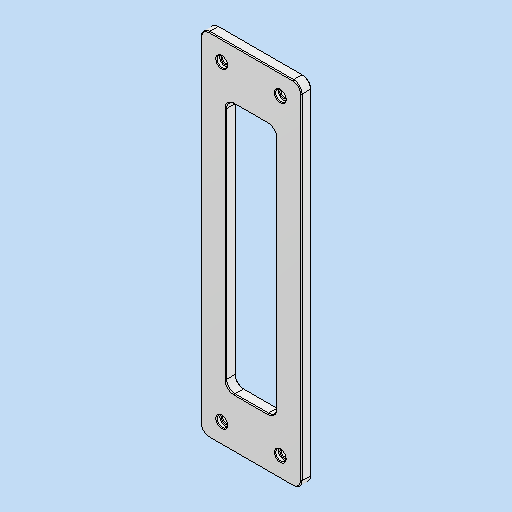
# Autodesk Inventor part: tc-top-bar
Saved by Autodesk Inventor 2026 (Build 300175050, 175E)
## iProperties
Created: 2025-06-05
Part Number: tc-top-bar
Material: ABS Plastic
Document SubType Name: Modeling
Designer: queezz
Density: 1.06 g/cm^3
Appearance: Smooth - White
Author: queezz
Autodesk Inventor part; units mm, degrees
ref_plane "YZ Plane" through (0, 0, 0) normal (1, 0, 0) x (0, 1, 0)
ref_plane "XZ Plane" through (0, 0, 0) normal (0, 1, 0) x (-1, 0, 0)
ref_plane "XY Plane" through (0, 0, 0) normal (0, 0, 1) x (1, 0, 0)
sketch "Sketch1" plane through (0, 0, 0) normal (0, 0, 1) x (1, 0, 0)
  line L0 (-30, 105) -> (30, 105)
  line L1 (30, 105) -> (30, -105)
  line L2 (30, -105) -> (-30, -105)
  line L3 (-30, -105) -> (-30, 105)
  point P0 (0, 0)
  point P1 (30, 0)
  point P2 (0, 105)
  dimension "d0" = 60
  dimension "d1" = 210
  constraints: 8 end point, 2 midpoint, 2 parallel, 1 horizontal, 1 horizontal alignment, 1 perpendicular, 1 vertical alignment
  measures "d0" distance of L0.start L0.end
  measures "d1" distance of L0.end L1.end
extrude "Extrusion1" add sketch "Sketch1" along normal blind 6
sketch "Sketch4" plane through (0, 0, 6) normal (0, 0, 1) x (1, 0, 0)
  line L0 (-15, 75) -> (15, 75)
  line L1 (15, 75) -> (15, -75)
  line L2 (15, -75) -> (-15, -75)
  line L3 (-15, -75) -> (-15, 75)
  line L4 (30, -105) -> (30, 105) projected
  line L5 (30, 105) -> (-30, 105) projected
  point P0 (0, 0)
  point P1 (0, 75)
  point P2 (15, 0)
  dimension "d20" = 15
  dimension "d21" = 30
  constraints: 8 end point, 2 midpoint, 2 parallel, 1 horizontal, 1 horizontal alignment, 1 perpendicular, 1 vertical alignment
  measures "d20" distance between parallel lines of L4 L1
  measures "d21" distance between parallel lines of L0 L5
extrude "Extrusion4" cut sketch "Sketch4" against normal through all
fillet "Fillet1" radius 5 8 edges at (-30, 105, 3) (30, 105, 3) (30, -105, 3) (-30, -105, 3) (-15, 75, 3) (15, 75, 3) (15, -75, 3) (-15, -75, 3)
chamfer "Chamfer2" distance 0.5 angle 45 32 edges at (0, 105, 6) (-28.5355, 103.5355, 6) (-30, 0, 6) (-28.5355, -103.5355, 6) (0, -105, 6) (28.5355, -103.5355, 6) (30, 0, 6) (28.5355, 103.5355, 6) (0, 105, 0) (-28.5355, 103.5355, 0) (-30, 0, 0) (-28.5355, -103.5355, 0) (0, -105, 0) (28.5355, -103.5355, 0) (30, 0, 0) (28.5355, 103.5355, 0) (-15, 0, 6) (-13.5355, 73.5355, 6) (0, 75, 6) (13.5355, 73.5355, 6) (15, 0, 6) (13.5355, -73.5355, 6) (0, -75, 6) (-13.5355, -73.5355, 6) (-15, 0, 0) (-13.5355, -73.5355, 0) (0, -75, 0) (13.5355, -73.5355, 0) (15, 0, 0) (13.5355, 73.5355, 0) (0, 75, 0) (-13.5355, 73.5355, 0)
sketch "Sketch5" plane through (0, 0, 6) normal (0, 0, 1) x (1, 0, 0)
  line L0 (-17.5, 93) -> (17.5, 93) construction
  line L1 (17.5, 93) -> (17.5, -93) construction
  line L2 (17.5, -93) -> (-17.5, -93) construction
  line L3 (-17.5, -93) -> (-17.5, 93) construction
  line L4 (25, 105) -> (-25, 105) construction
  point P0 (0, 0)
  point P1 (0, 93)
  point P2 (17.5, 0)
  point P3 (81.7088, -86.6952)
  dimension "d24" = 12
  dimension "d25" = 35
  constraints: 8 end point, 4 coincident, 2 midpoint, 2 parallel, 1 horizontal, 1 horizontal alignment, 1 perpendicular, 1 vertical alignment
  measures "d24" distance between parallel lines of L4 L0
  measures "d25" distance of L0.start L0.end
hole "Hole1" at (-17.5, 93, 6) at (17.5, 93, 6) at (17.5, -93, 6) at (-17.5, -93, 6) at (81.7088, -86.6952, 6) direction (0, 0, -1) diameter 3.6 end through all counterbore diameter 6.2 counterbore depth 2
chamfer "Chamfer3" distance 0.4 angle 45 12 edges at (17.5, -91.2, 0) (-17.5, -91.2, 0) (-17.5, 94.8, 0) (17.5, 94.8, 0) (17.5, 96.1, 6) (-17.5, 96.1, 6) (17.5, 94.8, 4) (-17.5, 94.8, 4) (-17.5, -89.9, 6) (-17.5, -91.2, 4) (17.5, -91.2, 4) (17.5, -89.9, 6)
equation "\"d0\" = width"
equation "\"d1\" = hight"
equation "\"hight\" = 210"
equation "\"width\" = 60"
body "Solid1"
